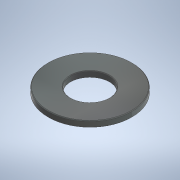
# Autodesk Inventor part: 3mm Rubber Washer
Saved by Autodesk Inventor 2021.1 (Build 251245010, 245A)
## iProperties
Created: 2025-09-16
Part Number: 3mm Rubber Washer
Material: Rubber
Document SubType Name: Modeling
Designer: SD
Density: 0.93 g/cm^3
Appearance: Rubble - River Rock
Mass: 0.014081 g
Surface Area: 0.750291 cm^2
Volume: 0.0151409 cm^3
Project: Automatic Tea Steeping mechanism
BOM-Mass: 0.00001
BOM-Area: 0.000
DateTimeString: 28-10-25 15:37
Date: 2025-10-28
Thickness: 0.500 mm
Diameter: 7.000 mm
Author: SD
Title: 3mm Rubber Washer
Autodesk Inventor part; units mm, degrees
ref_plane "YZ Plane" through (0, 0, 0) normal (1, 0, 0) x (0, 1, 0)
ref_plane "XZ Plane" through (0, 0, 0) normal (0, 1, 0) x (-1, 0, 0)
ref_plane "XY Plane" through (0, 0, 0) normal (0, 0, 1) x (1, 0, 0)
sketch "Sketch1" plane through (0, 0, 0) normal (0, 1, 0) x (-1, 0, 0)
  circle A0 centre (0, 0) radius 3.5
  circle A1 centre (0, 0) radius 1.6
  dimension "Diameter" = 7
  dimension "d1" = 3.2
  constraints: 2 centre point, 2 coincident
  measures "Diameter" diameter of A0
  measures "d1" diameter of A1
extrude "Extrusion1" add sketch "Sketch1" along normal blind 0.5
chamfer "Chamfer1" distance 0.05 angle 45 4 edges at (3.5, 0.5, 0) (1.6, 0.5, 0) (3.5, 0, 0) (1.6, 0, 0)
body "Solid1"
